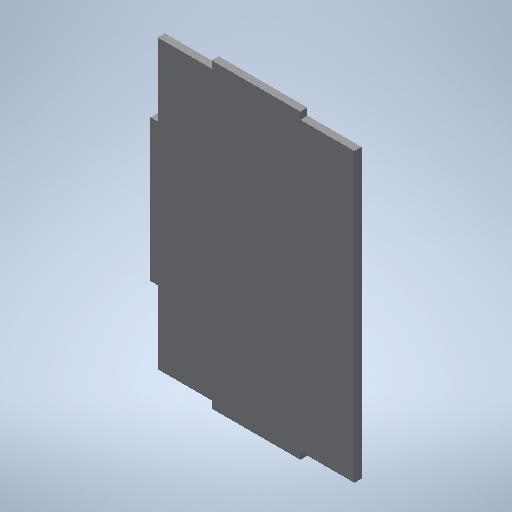
# Autodesk Inventor part: Tapa Superior
Saved by Autodesk Inventor 2025 (Build 290162000, 162)
## iProperties
Created: 2024-10-18
Part Number: Tapa Superior
Material: Generic
Document SubType Name: Modeling
Designer: feder
Density: 1 g/cm^3
Appearance: Default
Author: feder
Autodesk Inventor part; units mm, degrees
ref_plane "YZ Plane" through (0, 0, 0) normal (1, 0, 0) x (0, 1, 0)
ref_plane "XZ Plane" through (0, 0, 0) normal (0, 1, 0) x (-1, 0, 0)
ref_plane "XY Plane" through (0, 0, 0) normal (0, 0, 1) x (1, 0, 0)
sketch "Sketch1" plane through (0, 0, 0) normal (0, 0, 1) x (1, 0, 0)
  line L0 (-55.5, 81) -> (55.5, 81)
  line L1 (55.5, 81) -> (55.5, -81)
  line L2 (55.5, -81) -> (-55.5, -81)
  line L3 (-55.5, -81) -> (-55.5, 81)
  point P0 (0, 0)
  point P1 (55.5, 0)
  point P2 (0, -81)
  dimension "d0" = 111
  dimension "d1" = 162
  constraints: 8 end point, 2 midpoint, 2 parallel, 1 horizontal, 1 horizontal alignment, 1 perpendicular, 1 vertical alignment
  measures "d0" distance of L0.start L0.end
  measures "d1" distance of L0.end L1.end
extrude "Extrusion1" add sketch "Sketch1" along normal blind 4
sketch "Sketch2" plane through (-55.5, -81, 0) normal (-1, 0, 0) x (0, 0, 1)
  line L0 (4, 0) -> (4, 162) projected
  line L1 (0, 121) -> (4, 121)
  line L2 (4, 121) -> (4, 41)
  line L3 (4, 41) -> (0, 41)
  line L4 (0, 41) -> (0, 121)
  line L5 (0, 162) -> (0, 0) projected
  point P0 (0, 81)
  point P1 (0, 81)
  dimension "d4" = 80
  dimension "d5" = 40
  constraints: 8 end point, 2 parallel, 1 horizontal, 1 midpoint, 1 perpendicular, 1 point on line
  measures "d4" distance of L3.end L1.start
  measures "d5" distance from line of L1 point (0, 81)
extrude "Extrusion2" add sketch "Sketch2" along normal blind 4
sketch "Sketch3" plane through (-55.5, 81, 0) normal (0, 1, 0) x (1, 0, 0)
  line L0 (111, -4) -> (0, -4) projected
  line L1 (111, 0) -> (0, 0) projected
  line L2 (30.5, -4) -> (80.5, -4)
  line L3 (80.5, -4) -> (80.5, 0)
  line L4 (80.5, 0) -> (30.5, 0)
  line L5 (30.5, 0) -> (30.5, -4)
  point P0 (55.5, 0)
  point P1 (80.5, -2)
  point P2 (30.5, -2)
  point P3 (55.5, 0)
  point P4 (30.5, 0)
  dimension "d8" = 50
  dimension "d9" = 25
  constraints: 8 end point, 3 midpoint, 2 parallel, 2 point on line, 1 horizontal, 1 perpendicular
  measures "d8" distance of point (80.5, -2) point (30.5, -2)
  measures "d9" horizontal distance of point (30.5, -2) point (55.5, 0)
extrude "Extrusion3" add sketch "Sketch3" along normal blind 4
mirror "Mirror1" about plane through (0, 0, 0) normal (0, 1, 0) of "Extrusion3"
body "Solid1"
